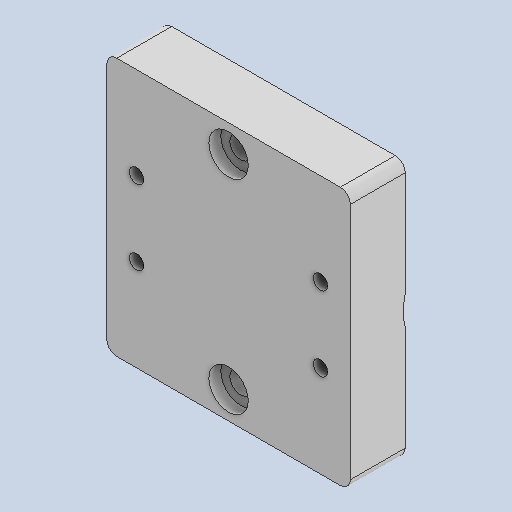
# Autodesk Inventor part: ADAPTER_EOM2.1GHz_new
Saved by Autodesk Inventor 2024.2 (Build 282272000, 272)
## iProperties
Created: 2021-07-16
Part Number: ADAPTER_EOM2.1GHz_new
Material: Generic
Document SubType Name: Modeling
Designer: paige
Density: 1 g/cm^3
Appearance: Default
Author: paige
Autodesk Inventor part; units mm, degrees
ref_plane "YZ Plane" through (0, 0, 0) normal (1, 0, 0) x (0, 1, 0)
ref_plane "XZ Plane" through (0, 0, 0) normal (0, 1, 0) x (-1, 0, 0)
ref_plane "XY Plane" through (0, 0, 0) normal (0, 0, 1) x (1, 0, 0)
sketch "Sketch1" plane through (0, 0, 0) normal (0, 0, 1) x (1, 0, 0)
  line L0 (-24.5, 26) -> (24.5, 26)
  line L1 (24.5, 26) -> (24.5, -26)
  line L2 (24.5, -26) -> (-24.5, -26)
  line L3 (-24.5, -26) -> (-24.5, 26)
  point P0 (0, 0)
  dimension "d0" = 52
  dimension "d1" = 26
  dimension "d2" = 49
  dimension "d3" = 24.5
  constraints: 8 end point, 2 parallel, 1 horizontal, 1 perpendicular
  measures "d0" distance of L2.end L0.start
  measures "d1" distance from line of L0 point (0, 0)
  measures "d2" distance of L1.end L2.end
  measures "d3" distance from line of L1 point (0, 0)
extrude "Extrusion1" add sketch "Sketch1" along normal blind 11.05
sketch "Sketch3" plane through (0, 0, 11.05) normal (0, 0, 1) x (1, 0, 0)
  line L0 (-24.5, -26) -> (24.5, -26) projected
  line L1 (0, -26) -> (0, -20.5)
  line L2 (24.5, 26) -> (-24.5, 26) projected
  line L3 (0, 26) -> (0, 20.5)
  point P0 (0, 0)
  point P1 (0, 0)
  dimension "d13" = 5.5
  dimension "d14" = 20.5
  dimension "d15" = 5.5
  dimension "d16" = 20.5
  constraints: 4 end point, 3 coincident, 2 midpoint, 2 vertical, 1 other
  measures "d13" distance of L1.start L1.end
  measures "d14" distance of point (0, 0) L1.end
  measures "d15" distance of L3.start L3.end
  measures "d16" distance of L3.end point (0, 0)
hole "Hole1" at (0, 20.5, 11.05) at (0, -20.5, 11.05) direction (0, 0, -1) diameter 4.305 depth 12.3 counterbore diameter 7.938 counterbore depth 2.4 clearance for "Socket Head Cap Screw" size "#8" standard "Ansi Unified Screw Threads"
fillet "Fillet1" radius 2 4 edges at (-24.5, -26, 5.525) (-24.5, 26, 5.525) (24.5, -26, 5.525) (24.5, 26, 5.525)
sketch "Sketch7" plane through (-24.5, -24, 0) normal (-1, 0, 0) x (0, 0, 1)
  circle A0 centre (-12.35, 24) radius 12.7
  point P0 (0, 24)
  dimension "d57" = 25.4
  dimension "d58" = 12.35
  constraints: 1 centre point
  measures "d57" diameter of A0
  measures "d58" distance of point (0, 24) A0.centre
extrude "Extrusion3" cut sketch "Sketch7" against normal blind 50
sketch "Sketch11" plane through (0, 0, 11.05) normal (0, 0, 1) x (1, 0, 0)
  line L0 (0, 0) -> (0, -15) construction
  line L1 (0, 0) -> (0, 15) construction
  line L2 (0, 0) -> (22.5, 0) construction
  line L3 (22.5, 0) -> (22.5, -15) construction
  line L4 (22.5, 0) -> (22.5, 15) construction
  line L5 (0, 0) -> (-22.5, 0) construction
  line L6 (-22.5, 0) -> (-22.5, -15) construction
  line L7 (-22.5, 0) -> (-22.5, 15) construction
  line L8 (22.5, -15) -> (-22.5, -15) construction
  line L9 (22.5, 15) -> (-22.5, 15) construction
  line L10 (-15.4375, 7.9375) -> (15.4375, 7.9375) construction
  line L11 (15.4375, -7.9375) -> (-15.4375, -7.9375) construction
  line L12 (-18.6125, -11.1125) -> (-18.6125, 0) construction
  line L13 (-18.6125, 0) -> (-18.6125, 11.1125) construction
  line L14 (18.6125, 11.1125) -> (18.6125, 0) construction
  line L15 (18.6125, 0) -> (18.6125, -11.1125) construction
  line L16 (15.4375, -7.9375) -> (18.6125, -7.9375) construction
  line L17 (15.4375, 7.9375) -> (18.6125, 7.9375) construction
  line L18 (-15.4375, -7.9375) -> (-18.6125, -7.9375) construction
  line L19 (-15.4375, 7.9375) -> (-18.6125, 7.9375) construction
  line L20 (18.6125, -7.9375) -> (29.1538, -7.9375) construction
  line L21 (18.6125, 7.9375) -> (28.0959, 7.9375) construction
  line L22 (-18.6125, -7.9375) -> (-33.3375, -7.9375) construction
  line L23 (-18.6125, 7.9375) -> (-34.925, 7.9375) construction
  dimension "d98" = 22.5
  dimension "d99" = 15
  dimension "d100" = 15
  dimension "d101" = 22.5
  dimension "d102" = 15
  dimension "d103" = 15
  dimension "d104" = 7.0625
  constraints: 48 end point, 8 horizontal, 5 vertical, 4 point on line, 2 other
  measures "d98" distance of L0.start L2.end
  measures "d99" distance of L2.end L3.end
  measures "d100" distance of L2.end L4.end
  measures "d101" distance of L0.start L5.end
  measures "d102" distance of L5.end L6.end
  measures "d103" distance of L5.end L7.end
  measures "d104" distance between parallel lines of L8 L11
hole "Hole6" [suppressed]
sketch "Sketch12" plane through (0, 0, 0) normal (0, 0, -1) x (-1, 0, 0)
  line L0 (-22.5, 0) -> (-22.5, 15) construction
  line L1 (22.5, 0) -> (22.5, 15) construction
  line L2 (-22.5, 0) -> (-22.5, -15) construction
  line L3 (22.5, 0) -> (22.5, -15) construction
  line L4 (24.5, 24) -> (24.5, -24) construction
  line L5 (-22.5, 15) -> (22.5, 15) construction
  line L6 (-22.5, -15) -> (22.5, -15) construction
  line L7 (-18.5, 11.55) -> (-18.5, 0) construction
  line L8 (-18.5, 0) -> (-18.5, -11.55) construction
  line L9 (18.5, -11.55) -> (18.5, 0) construction
  line L10 (18.5, 0) -> (18.5, 11.55) construction
  line L11 (15.9875, -7.5) -> (-14.8875, -7.5) construction
  line L12 (-15.4375, 7.5) -> (15.4375, 7.5) construction
  line L13 (-15.4375, 7.5) -> (-18.5, 7.5) construction
  line L14 (15.4375, 7.5) -> (18.5, 7.5) construction
  line L15 (-14.8875, -7.5) -> (-18.5, -7.5) construction
  line L16 (15.9875, -7.5) -> (18.5, -7.5) construction
  line L17 (-18.5, 7.5) -> (-21.7329, 7.5) construction
  line L18 (-18.5, -7.5) -> (-20.6685, -7.5) construction
  line L19 (18.5, -7.5) -> (22.1748, -7.5) construction
  line L20 (18.5, 7.5) -> (20.6375, 7.5) construction
  point P0 (0, 0)
  dimension "d115" = 15
  dimension "d117" = 4
  dimension "d118" = 7.5
  dimension "d126" = 45
  dimension "d127" = 15
  dimension "d128" = 4
  dimension "d129" = 7.5
  constraints: 40 end point, 4 horizontal, 4 perpendicular, 4 point on line, 2 vertical, 2 other
  measures "d115" distance of L0.start L0.end
  measures "d117" distance between parallel lines of L0 L7
  measures "d118" distance between parallel lines of L5 L12
  measures "d126" distance of L2.end L3.end
  measures "d127" distance of L0.start L2.end
  measures "d128" distance between parallel lines of L3 L9
  measures "d129" distance between parallel lines of L11 L6
hole "Hole7" at (18.5, 7.5, 0) at (-18.5, 7.5, 0) at (18.5, -7.5, 0) at (-18.5, -7.5, 0) direction (0, 0, 1) diameter 2.9 end through all counterbore diameter 5.5 counterbore depth 2.5 clearance for "Socket Head Cap Screw" size "M2.5" standard "Ansi Metric M Profile"
equation "\"d1\" = 0.5 * d0"
equation "\"d3\" = 0.5 * d2"
equation "\"d15\" = d13"
body "Solid1"
